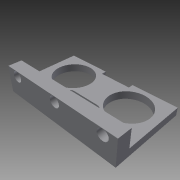
# Autodesk Inventor part: Mount for US
Saved by Autodesk Inventor 2015 (Build 190159000, 159)
## iProperties
Created: 2018-11-11
Part Number: Mount for US
Material: Типовые
Document SubType Name: Modeling
Designer: kostya
Density: 1 g/cm^3
Appearance: По умолчанию
Author: kostya
Autodesk Inventor part; units mm, degrees
ref_plane "YZ Plane" through (0, 0, 0) normal (1, 0, 0) x (0, 1, 0)
ref_plane "XZ Plane" through (0, 0, 0) normal (0, 1, 0) x (-1, 0, 0)
ref_plane "XY Plane" through (0, 0, 0) normal (0, 0, 1) x (1, 0, 0)
sketch "Эскиз3" plane through (0, 0, 0) normal (0, 0, 1) x (1, 0, 0)
  line L0 (22.95, -10.5) -> (22.95, 10.5)
  line L1 (-22.95, 10.5) -> (-22.95, -10.5)
  line L2 (-22.95, -10.5) -> (22.95, 10.5) construction
  line L3 (22.95, -10.5) -> (-22.95, 10.5) construction
  line L4 (-6, 10.5) -> (-22.95, 10.5) construction
  line L5 (6, 10.5) -> (22.95, 10.5) construction
  line L6 (22.95, 0) -> (19.95, 0) construction
  line L7 (16.3868, 10.5) -> (16.3868, 8.5) construction
  line L8 (17.599, 8.5) -> (14.8742, 8.5) construction
  line L9 (19.95, 1.7069) -> (19.95, -1.7382) construction
  line L10 (16.2366, -10.5) -> (16.2366, -7) construction
  line L11 (17.599, -7) -> (14.2766, -7) construction
  circle A0 centre (12.2, 0.75) radius 7.75
  line L12 (0, 10.5) -> (0, -10.5) construction
  line L13 (-22.95, 0) -> (-19.95, 0) construction
  line L14 (-16.3868, 10.5) -> (-16.3868, 8.5) construction
  line L15 (-17.599, 8.5) -> (-14.8742, 8.5) construction
  line L16 (-19.95, 1.7069) -> (-19.95, -1.7382) construction
  line L17 (-16.2366, -10.5) -> (-16.2366, -7) construction
  line L18 (-17.599, -7) -> (-14.2766, -7) construction
  circle A1 centre (-12.2, 0.75) radius 7.75
  line L19 (-22.95, 0) -> (22.95, 0) construction
  line L20 (0, 8.5) -> (0, -5.5) construction
  line L21 (0, -5.5) -> (5, -5.5)
  line L22 (0, -5.5) -> (-5, -5.5)
  line L23 (-5, -10.5) -> (5, -10.5)
  arc A2 (-5, -5.5) -> (-5, -10.5) centre (-5, -8) ccw
  arc A3 (5, -10.5) -> (5, -5.5) centre (5, -8) ccw
  line L24 (-22.95, -10.5) -> (-22.95, -12.5)
  line L25 (-22.95, -12.5) -> (22.95, -12.5)
  line L26 (22.95, -12.5) -> (22.95, -10.5)
  line L27 (0, 8.5) -> (6, 8.5)
  line L28 (0, 8.5) -> (-6, 8.5)
  line L29 (-6, 8.5) -> (-6, 10.5)
  line L30 (6, 8.5) -> (6, 10.5)
  line L31 (22.95, 10.5) -> (6, 10.5)
  line L32 (-6, 10.5) -> (-22.95, 10.5)
  point P0 (0, 0)
  point P1 (5, -5.5)
  point P2 (-5, -5.5)
  dimension "d23" = 45.9
  dimension "d24" = 21
  dimension "d26" = 3
  dimension "d27" = 2
  dimension "d29" = 3.5
  dimension "d30" = 16
  dimension "d31" = 5
  dimension "d32" = 2.5
  dimension "d35" = 2
  dimension "d47" = 6
  dimension "d48" = 6
  constraints: 66 end point, 14 symmetric about line, 9 horizontal, 7 tangent, 5 equal length, 5 perpendicular, 4 centre point, 4 point on circle, 4 point on line, 3 midpoint, 3 vertical, 1 equal radius, 1 other
  measures "d23" distance of L1.start L0.end
  measures "d24" distance of L0.end L0.start
  measures "d26" distance of L6.start L6.end
  measures "d27" distance of L7.start L7.end
  measures "d29" distance of L10.start L10.end
  measures "d30" distance of L12.start L20.end
  measures "d31" distance of L20.end point (5, -5.5)
  measures "d32" radius of A2
  measures "d35" distance of L1.end L24.end
  measures "d47" distance of L20.start L27.end
  measures "d48" distance of L20.start L28.end
extrude "Выдавливание5" add sketch "Эскиз3" against normal blind 3
sketch "Эскиз4" plane through (0, 0, 0) normal (0, 0, 1) x (1, 0, 0)
  line L0 (-22.95, -12.5) -> (22.95, -12.5)
  line L1 (22.95, -12.5) -> (22.95, -17.5)
  line L2 (22.95, -17.5) -> (-22.95, -17.5)
  line L3 (-22.95, -17.5) -> (-22.95, -12.5)
  line L4 (22.95, -12.5) -> (-22.95, -12.5) projected
  point P0 (0, 0)
  dimension "d36" = 5
  constraints: 8 end point, 3 equal length, 1 perpendicular
  measures "d36" distance of L0.end L1.end
extrude "Выдавливание6" add sketch "Эскиз4" along normal blind 7 and the other way blind 3
sketch "Эскиз6" plane through (-22.95, -12.5, 0) normal (0, 1, 0) x (1, 0, 0)
  line L0 (45.9, 0) -> (0, 0) projected
  line L1 (0, -7) -> (0, 0) projected
  line L2 (45.9, -7) -> (0, -7) projected
  line L3 (45.9, 0) -> (45.9, -7) projected
  line L4 (45.9, 0) -> (45.9, -7) construction
  line L5 (45.9, -3.5) -> (0, -3.5) construction
  line L6 (0, -7) -> (0, 0) construction
  line L7 (0, -7) -> (45.9, -7) construction
  line L8 (22.95, -7) -> (22.95, 0) construction
  circle A0 centre (41.2273, -4.9258) radius 2
  circle A1 centre (4.6727, -4.9258) radius 2
  line L9 (45.9, -4.1809) -> (0, -4.1809) construction
  circle A2 centre (22.95, -4.9258) radius 2
  dimension "d50" = 4
  constraints: 6 end point, 3 centre point, 3 midpoint, 1 perpendicular, 1 vertical
  measures "d50" diameter of A0
extrude "Выдавливание8" cut sketch "Эскиз6" against normal blind 10 contours A0 | A1 | A2
